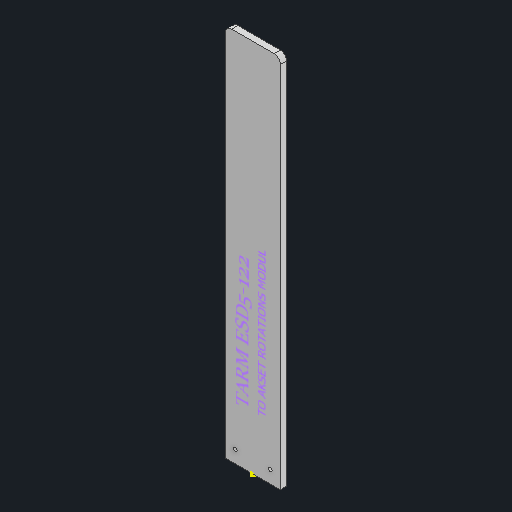
# Autodesk Inventor part: LEG
Saved by Autodesk Inventor 2023.4 (Build 274418000, 418)
## iProperties
Created: 2025-10-08
Part Number: LEG
Material: Generic
Document SubType Name: Modeling
Designer: Malthe Sennels
Density: 1 g/cm^3
Appearance: Default
Author: Malthe Sennels
Autodesk Inventor part; units mm, degrees
ref_plane "YZ Plane" through (0, 0, 0) normal (1, 0, 0) x (0, 1, 0)
ref_plane "XZ Plane" through (0, 0, 0) normal (0, 1, 0) x (-1, 0, 0)
ref_plane "XY Plane" through (0, 0, 0) normal (0, 0, 1) x (1, 0, 0)
sketch "Sketch1" plane through (0, 0, 0) normal (0, 0, 1) x (1, 0, 0)
  line L0 (-22, 20.2116) -> (-22, 0.2116) projected
  line L1 (22, 0.2116) -> (-22, 0.2116) projected
  line L2 (22, 0.2116) -> (22, 20.2116) projected
  line L3 (-22, 20.2116) -> (22, 20.2116) projected
  line L4 (22, 0.2116) -> (-22, 0.2116)
  line L5 (-22, 0.2116) -> (-22, 295.2116)
  line L6 (-17, 300.2116) -> (17, 300.2116)
  line L7 (22, 295.2116) -> (22, 0.2116)
  arc A0 (22, 295.2116) -> (17, 300.2116) centre (17, 295.2116) ccw
  arc A1 (-17, 300.2116) -> (-22, 295.2116) centre (-17, 295.2116) ccw
  circle A2 centre (14, 10.2116) radius 1.5
  line L8 (0, 0) -> (0, 26.7557)
  circle A3 centre (-14, 10.2116) radius 1.5
  circle A4 centre (-14, 10.2116) radius 1.5 projected
  circle A5 centre (14, 10.2116) radius 1.5 projected
  point P0 (-22, 300.2116)
  dimension "d0" = 300
  dimension "d1" = 5
  dimension "d2" = 3
  dimension "d3" = 14
  dimension "d4" = 10
  constraints: 10 end point, 4 centre point, 4 point on circle, 4 tangent, 3 point on line, 2 parallel, 1 equal radius, 1 horizontal, 1 perpendicular, 1 symmetric about line, 1 vertical, 2 other
  measures "d0" distance of L4.end point (-22, 300.212)
  measures "d1" radius of A0
  measures "d2" diameter of A2
  measures "d3" distance from line of A2.centre L8
extrude "Extrusion1" add sketch "Sketch1" along normal blind 5
sketch "Sketch2" plane through (0, 0, 5) normal (0, 0, 1) x (1, 0, 0)
  line L0 (-13.8628, 42.4038) -> (-13.8628, 167.0057) construction
  line L1 (-13.8628, 167.0057) -> (11.2533, 167.0057) construction
  line L2 (11.2533, 167.0057) -> (11.2533, 42.4038) construction
  line L3 (11.2533, 42.4038) -> (-13.8628, 42.4038) construction
  line L4 (3.9056, 43.7737) -> (3.9056, 205.2342) construction
  line L5 (3.9056, 205.2342) -> (61.2284, 205.2342) construction
  line L6 (61.2284, 205.2342) -> (61.2284, 43.7737) construction
  line L7 (61.2284, 43.7737) -> (3.9056, 43.7737) construction
  point P0 (0, 0)
  constraints: 4 other
body "Solid1"
